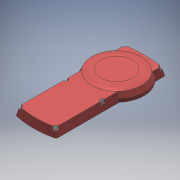
# Autodesk Inventor part: ET8
Saved by Autodesk Inventor 2016 (Build 200138000, 138)
## iProperties
Created: 2016-03-20
Part Number: ET8
Material: Genérico
Document SubType Name: Modeling
Designer: Usuario1
Density: 1 g/cm^3
Appearance: Valor por defecto
Author: Usuario1
Autodesk Inventor part; units mm, degrees
ref_plane "YZ Plane" through (0, 0, 0) normal (1, 0, 0) x (0, 1, 0)
ref_plane "XZ Plane" through (0, 0, 0) normal (0, 1, 0) x (-1, 0, 0)
ref_plane "XY Plane" through (0, 0, 0) normal (0, 0, 1) x (1, 0, 0)
sketch "Boceto1" plane through (0, 0, 0) normal (0, 0, 1) x (1, 0, 0)
  arc A0 (0.1163, -0.2747) -> (3.2914, -0.2747) centre (1.7039, 6.6157) ccw
  arc A1 (3.2914, -0.2747) -> (3.4078, -0.1285) centre (3.2578, -0.1285) ccw
  arc A2 (0, -0.1285) -> (0.1163, -0.2747) centre (0.15, -0.1285) ccw
  circle A3 centre (1.7039, 6.4933) radius 2.0393
  circle A4 centre (0.1483, 3.7581) radius 0.092
  arc A5 (3.2776, 8.8751) -> (0.1302, 8.8751) centre (1.7039, -2.9316) ccw
  arc A6 (3.4078, 8.7264) -> (3.2776, 8.8751) centre (3.2578, 8.7264) ccw
  arc A7 (0.1302, 8.8751) -> (0, 8.7264) centre (0.15, 8.7264) ccw
  line L0 (0, 3.6296) -> (0.16, 3.6296)
  arc A8 (0.16, 3.6296) -> (0.28, 3.7496) centre (0.16, 3.7496) ccw
  line L1 (0.28, 3.7496) -> (0.28, 3.7683)
  arc A9 (0.28, 3.7683) -> (0.16, 3.8883) centre (0.16, 3.7683) ccw
  line L2 (0.16, 3.8883) -> (0, 3.8883)
  circle A10 centre (0.15, 8.7264) radius 0.092
  line L3 (0, 8.5978) -> (0.16, 8.5978)
  line L4 (0.28, 8.8941) -> (0.28, 8.7178)
  arc A11 (0.16, 8.5978) -> (0.28, 8.7178) centre (0.16, 8.7178) ccw
  circle A12 centre (0.15, -0.1285) radius 0.092
  line L5 (0, 0) -> (0.16, 0)
  line L6 (0.28, -0.3104) -> (0.28, -0.12)
  arc A13 (0.28, -0.12) -> (0.16, 0) centre (0.16, -0.12) ccw
  circle A14 centre (3.2594, 3.7581) radius 0.092
  line L7 (3.4078, 3.6296) -> (3.2478, 3.6296)
  arc A15 (3.1278, 3.7496) -> (3.2478, 3.6296) centre (3.2478, 3.7496) ccw
  line L8 (3.1278, 3.7496) -> (3.1278, 3.7683)
  arc A16 (3.2478, 3.8883) -> (3.1278, 3.7683) centre (3.2478, 3.7683) ccw
  line L9 (3.2478, 3.8883) -> (3.4078, 3.8883)
  circle A17 centre (3.2578, 8.7264) radius 0.092
  line L10 (3.4078, 8.5978) -> (3.2478, 8.5978)
  line L11 (3.1278, 8.8941) -> (3.1278, 8.7178)
  arc A18 (3.1278, 8.7178) -> (3.2478, 8.5978) centre (3.2478, 8.7178) ccw
  circle A19 centre (3.2578, -0.1285) radius 0.092
  line L12 (3.4078, 0) -> (3.2478, 0)
  line L13 (3.1278, -0.3104) -> (3.1278, -0.12)
  arc A20 (3.2478, 0) -> (3.1278, -0.12) centre (3.2478, -0.12) ccw
  line L14 (0, 8.7264) -> (0, 7.9849)
  line L15 (3.4078, 8.7264) -> (3.4078, 7.9849)
  line L16 (0, 5.0017) -> (0, -0.1285)
  line L17 (3.4078, -0.1285) -> (3.4078, 5.0017)
  arc A21 (0, 7.9849) -> (0, 5.0017) centre (1.7039, 6.4933) ccw
  arc A22 (3.4078, 5.0017) -> (3.4078, 7.9849) centre (1.7039, 6.4933) ccw
  point P0 (0, 0)
  constraints: 36 end point, 36 point on circle, 23 centre point, 8 point on line
extrude "Extrusión1" add sketch "Boceto1" along normal blind 0.15 contours L6 A13 L5 L16 L0 A8 L1 A9 L2 A21 L14 L3 A11 L4 A5 L11 A18 L10 L15 A22 L17 L9 A16 L8 A15 L7 L12 A20 L13 A0 | A3
sketch "Boceto4" plane through (0, 0, 0) normal (0, 0, -1) x (-1, 0, 0)
  line L0 (0, 3.6296) -> (0, 0) projected
  line L1 (-0.16, 3.6296) -> (0, 3.6296) projected
  arc A0 (-0.28, 3.7496) -> (-0.16, 3.6296) centre (-0.16, 3.7496) ccw projected
  line L2 (-0.28, 3.7683) -> (-0.28, 3.7496) projected
  arc A1 (-0.16, 3.8883) -> (-0.28, 3.7683) centre (-0.16, 3.7683) ccw projected
  line L3 (0, 3.8883) -> (-0.16, 3.8883) projected
  line L4 (0, 5.0017) -> (0, 3.8883) projected
  arc A2 (0, 5.0017) -> (0, 7.9849) centre (-1.7039, 6.4933) ccw projected
  line L5 (0, 8.5978) -> (0, 7.9849) projected
  line L6 (-0.16, 8.5978) -> (0, 8.5978) projected
  arc A3 (-0.28, 8.7178) -> (-0.16, 8.5978) centre (-0.16, 8.7178) ccw projected
  line L7 (-0.28, 8.8941) -> (-0.28, 8.7178) projected
  arc A4 (-0.28, 8.8941) -> (-3.1278, 8.8941) centre (-1.7039, -2.9316) ccw projected
  line L8 (-3.1278, 8.7178) -> (-3.1278, 8.8941) projected
  arc A5 (-3.2478, 8.5978) -> (-3.1278, 8.7178) centre (-3.2478, 8.7178) ccw projected
  line L9 (-3.4078, 8.5978) -> (-3.2478, 8.5978) projected
  line L10 (-3.4078, 7.9849) -> (-3.4078, 8.5978) projected
  arc A6 (-3.4078, 7.9849) -> (-3.4078, 5.0017) centre (-1.7039, 6.4933) ccw projected
  line L11 (-3.4078, 3.8883) -> (-3.4078, 5.0017) projected
  line L12 (-3.2478, 3.8883) -> (-3.4078, 3.8883) projected
  arc A7 (-3.1278, 3.7683) -> (-3.2478, 3.8883) centre (-3.2478, 3.7683) ccw projected
  line L13 (-3.1278, 3.7496) -> (-3.1278, 3.7683) projected
  arc A8 (-3.2478, 3.6296) -> (-3.1278, 3.7496) centre (-3.2478, 3.7496) ccw projected
  line L14 (-3.4078, 3.6296) -> (-3.2478, 3.6296) projected
  line L15 (-3.4078, 0) -> (-3.4078, 3.6296) projected
  line L16 (-3.2478, 0) -> (-3.4078, 0) projected
  arc A9 (-3.1278, -0.12) -> (-3.2478, 0) centre (-3.2478, -0.12) ccw projected
  line L17 (-3.1278, -0.3104) -> (-3.1278, -0.12) projected
  arc A10 (-3.1278, -0.3104) -> (-0.28, -0.3104) centre (-1.7039, 6.6157) ccw projected
  line L18 (-0.28, -0.12) -> (-0.28, -0.3104) projected
  arc A11 (-0.16, 0) -> (-0.28, -0.12) centre (-0.16, -0.12) ccw projected
  line L19 (0, 0) -> (-0.16, 0) projected
  arc A12 (-0.5269, 8.6699) -> (-2.8809, 8.6699) centre (-1.7039, -2.9316) ccw
  arc A13 (-0.5269, 8.6699) -> (-0.25, 8.359) centre (-0.16, 8.7178) ccw
  line L20 (-0.25, 8.359) -> (-0.25, 7.8877)
  arc A14 (-0.25, 5.0988) -> (-0.25, 7.8877) centre (-1.7039, 6.4933) ccw
  line L21 (-0.25, 5.0988) -> (-0.25, 4.1271)
  arc A15 (-0.25, 4.1271) -> (-0.53, 3.7683) centre (-0.16, 3.7683) ccw
  line L22 (-0.53, 3.7683) -> (-0.53, 3.7496)
  arc A16 (-0.53, 3.7496) -> (-0.25, 3.3907) centre (-0.16, 3.7496) ccw
  line L23 (-0.25, 3.3907) -> (-0.25, 0.2389)
  arc A17 (-0.25, 0.2389) -> (-0.5296, -0.1034) centre (-0.16, -0.12) ccw
  arc A18 (-2.8781, -0.1034) -> (-0.5296, -0.1034) centre (-1.7039, 6.6157) ccw
  arc A19 (-2.8781, -0.1034) -> (-3.1578, 0.2389) centre (-3.2478, -0.12) ccw
  line L24 (-3.1578, 0.2389) -> (-3.1578, 3.3907)
  arc A20 (-3.1578, 3.3907) -> (-2.8778, 3.7496) centre (-3.2478, 3.7496) ccw
  line L25 (-2.8778, 3.7496) -> (-2.8778, 3.7683)
  arc A21 (-2.8778, 3.7683) -> (-3.1578, 4.1271) centre (-3.2478, 3.7683) ccw
  line L26 (-3.1578, 4.1271) -> (-3.1578, 5.0988)
  arc A22 (-3.1578, 7.8877) -> (-3.1578, 5.0988) centre (-1.7039, 6.4933) ccw
  line L27 (-3.1578, 7.8877) -> (-3.1578, 8.359)
  arc A23 (-3.1578, 8.359) -> (-2.8809, 8.6699) centre (-3.2478, 8.7178) ccw
  point P0 (0, 0)
  dimension "d10" = 0.25
  constraints: 24 point on circle, 16 end point, 12 centre point, 19 other
  measures "d10" radial gap between concentric circles of A4 A12
extrude "Extrusión4" add sketch "Boceto4" along normal blind 0.52
sketch "Boceto5" plane through (0, 0, 0.15) normal (0, 0, 1) x (1, 0, 0)
  arc A0 (3.2202, 5.0739) -> (3.2202, 7.9126) centre (1.7039, 6.4933) ccw projected
  circle A1 centre (1.7039, 6.4933) radius 2.077
  point P0 (0, 0)
  constraints: 1 coincident, 3 other
extrude "Extrusión5" add sketch "Boceto5" along normal blind 0.15
fillet "Empalme2" radius 2 1 edges at (-0.3731, 6.4933, 0.3)
chamfer "Chaflán12" distance 0.67 angle 15 1 edges at (0, 4.445, 0.15) measured on face at (0, 4.445, -0.35)
chamfer "Chaflán13" distance 0.67 angle 15 1 edges at (0, 1.8148, 0.15) measured on face at (0, 1.8148, -0.35)
chamfer "Chaflán14" distance 0.67 angle 15 1 edges at (1.7039, -0.4552, 0.15) measured on face at (1.7039, -0.4552, -0.35)
chamfer "Chaflán15" distance 0.67 angle 15 1 edges at (3.4078, 1.8148, 0.15) measured on face at (3.4078, 1.8148, -0.35)
chamfer "Chaflán16" distance 0.67 angle 15 1 edges at (3.4078, 4.445, 0.15) measured on face at (3.4078, 4.445, -0.35)
chamfer "Chaflán17" distance 0.67 angle 15 1 edges at (1.7039, 8.9795, 0.15) measured on face at (1.7039, 8.9795, -0.35)
chamfer "Chaflán18" distance 0.67 angle 15 1 edges at (3.4078, 8.2914, 0.15) measured on face at (3.4078, 8.2914, -0.35)
chamfer "Chaflán19" distance 0.67 angle 15 1 edges at (0, 8.2914, 0.15) measured on face at (0, 8.2914, -0.35)
chamfer "Chaflán20" distance 0.4 angle 25 3 edges at (3.3206, 8.0789, 0.15) (3.9684, 6.4933, 0.15) (3.3206, 4.9077, 0.15) measured on face at (3.3206, 8.0789, 0.05) measured on face at (3.3206, 4.9077, 0.05) measured on face at (3.9684, 6.4933, -0.35)
chamfer "Chaflán21" distance 0.4 angle 25 3 edges at (0.0871, 8.0789, 0.15) (-0.5606, 6.4933, 0.15) (0.0871, 4.9077, 0.15) measured on face at (-0.5606, 6.4933, -0.35) measured on face at (0.0871, 8.0789, 0.05) measured on face at (0.0871, 4.9077, 0.05)
sketch "Boceto8" plane through (0, 0, -0.52) normal (0, 0, -1) x (-1, 0, 0)
  arc A0 (-0.5269, 8.6699) -> (-0.25, 8.359) centre (-0.16, 8.7178) ccw projected
  line L0 (-0.25, 8.359) -> (-0.25, 7.8877) projected
  arc A1 (-0.25, 5.0988) -> (-0.25, 7.8877) centre (-1.7039, 6.4933) ccw projected
  line L1 (-0.25, 5.0988) -> (-0.25, 4.1271) projected
  arc A2 (-0.25, 4.1271) -> (-0.53, 3.7683) centre (-0.16, 3.7683) ccw projected
  line L2 (-0.53, 3.7683) -> (-0.53, 3.7496) projected
  arc A3 (-0.53, 3.7496) -> (-0.25, 3.3907) centre (-0.16, 3.7496) ccw projected
  line L3 (-0.25, 3.3907) -> (-0.25, 0.2389) projected
  arc A4 (-0.25, 0.2389) -> (-0.5296, -0.1034) centre (-0.16, -0.12) ccw projected
  arc A5 (-2.8781, -0.1034) -> (-0.5296, -0.1034) centre (-1.7039, 6.6157) ccw projected
  arc A6 (-2.8781, -0.1034) -> (-3.1578, 0.2389) centre (-3.2478, -0.12) ccw projected
  line L4 (-3.1578, 0.2389) -> (-3.1578, 3.3907) projected
  arc A7 (-3.1578, 3.3907) -> (-2.8778, 3.7496) centre (-3.2478, 3.7496) ccw projected
  line L5 (-2.8778, 3.7496) -> (-2.8778, 3.7683) projected
  arc A8 (-2.8778, 3.7683) -> (-3.1578, 4.1271) centre (-3.2478, 3.7683) ccw projected
  line L6 (-3.1578, 4.1271) -> (-3.1578, 5.0988) projected
  arc A9 (-3.1578, 7.8877) -> (-3.1578, 5.0988) centre (-1.7039, 6.4933) ccw projected
  line L7 (-3.1578, 7.8877) -> (-3.1578, 8.359) projected
  arc A10 (-3.1578, 8.359) -> (-2.8809, 8.6699) centre (-3.2478, 8.7178) ccw projected
  arc A11 (-0.5269, 8.6699) -> (-2.8809, 8.6699) centre (-1.7039, -2.9316) ccw projected
  line L8 (0, 0) -> (0, 3.6296) projected
  line L9 (0, 3.6296) -> (-0.16, 3.6296) projected
  arc A12 (-0.28, 3.7496) -> (-0.16, 3.6296) centre (-0.16, 3.7496) ccw projected
  line L10 (-0.28, 3.7496) -> (-0.28, 3.7683) projected
  arc A13 (-0.16, 3.8883) -> (-0.28, 3.7683) centre (-0.16, 3.7683) ccw projected
  line L11 (-0.16, 3.8883) -> (0, 3.8883) projected
  line L12 (0, 3.8883) -> (0, 5.0017) projected
  arc A14 (0, 5.0017) -> (0, 7.9849) centre (-1.7039, 6.4933) ccw projected
  line L13 (0, 7.9849) -> (0, 8.5978) projected
  line L14 (0, 8.5978) -> (-0.16, 8.5978) projected
  arc A15 (-0.28, 8.7178) -> (-0.16, 8.5978) centre (-0.16, 8.7178) ccw projected
  line L15 (-0.28, 8.7178) -> (-0.28, 8.8941) projected
  arc A16 (-0.28, 8.8941) -> (-3.1278, 8.8941) centre (-1.7039, -2.9316) ccw projected
  line L16 (-3.1278, 8.8941) -> (-3.1278, 8.7178) projected
  arc A17 (-3.2478, 8.5978) -> (-3.1278, 8.7178) centre (-3.2478, 8.7178) ccw projected
  line L17 (-3.2478, 8.5978) -> (-3.4078, 8.5978) projected
  line L18 (-3.4078, 8.5978) -> (-3.4078, 7.9849) projected
  arc A18 (-3.4078, 7.9849) -> (-3.4078, 5.0017) centre (-1.7039, 6.4933) ccw projected
  line L19 (-3.4078, 5.0017) -> (-3.4078, 3.8883) projected
  line L20 (-3.4078, 3.8883) -> (-3.2478, 3.8883) projected
  arc A19 (-3.1278, 3.7683) -> (-3.2478, 3.8883) centre (-3.2478, 3.7683) ccw projected
  line L21 (-3.1278, 3.7683) -> (-3.1278, 3.7496) projected
  arc A20 (-3.2478, 3.6296) -> (-3.1278, 3.7496) centre (-3.2478, 3.7496) ccw projected
  line L22 (-3.2478, 3.6296) -> (-3.4078, 3.6296) projected
  line L23 (-3.4078, 3.6296) -> (-3.4078, 0) projected
  line L24 (-3.4078, 0) -> (-3.2478, 0) projected
  arc A21 (-3.1278, -0.12) -> (-3.2478, 0) centre (-3.2478, -0.12) ccw projected
  line L25 (-3.1278, -0.12) -> (-3.1278, -0.3104) projected
  arc A22 (-3.1278, -0.3104) -> (-0.28, -0.3104) centre (-1.7039, 6.6157) ccw projected
  line L26 (-0.28, -0.3104) -> (-0.28, -0.12) projected
  arc A23 (-0.16, 0) -> (-0.28, -0.12) centre (-0.16, -0.12) ccw projected
  line L27 (-0.16, 0) -> (0, 0) projected
  arc A24 (-3.2914, -0.2747) -> (-0.1163, -0.2747) centre (-1.7039, 6.6157) ccw
  arc A25 (-0.1163, -0.2747) -> (0, -0.1285) centre (-0.15, -0.1285) ccw
  arc A26 (-3.4078, -0.1285) -> (-3.2914, -0.2747) centre (-3.2578, -0.1285) ccw
  circle A27 centre (-1.7039, 6.4933) radius 2.0393
  circle A28 centre (-3.2594, 3.7581) radius 0.092
  arc A29 (-0.1302, 8.8751) -> (-3.2776, 8.8751) centre (-1.7039, -2.9316) ccw
  arc A30 (0, 8.7264) -> (-0.1302, 8.8751) centre (-0.15, 8.7264) ccw
  arc A31 (-3.2776, 8.8751) -> (-3.4078, 8.7264) centre (-3.2578, 8.7264) ccw
  line L28 (-3.4078, 3.6296) -> (-3.2478, 3.6296)
  arc A32 (-3.2478, 3.6296) -> (-3.1278, 3.7496) centre (-3.2478, 3.7496) ccw
  line L29 (-3.1278, 3.7496) -> (-3.1278, 3.7683)
  arc A33 (-3.1278, 3.7683) -> (-3.2478, 3.8883) centre (-3.2478, 3.7683) ccw
  line L30 (-3.2478, 3.8883) -> (-3.4078, 3.8883)
  circle A34 centre (-3.2578, 8.7264) radius 0.092
  line L31 (-3.4078, 8.5978) -> (-3.2478, 8.5978)
  line L32 (-3.1278, 8.8941) -> (-3.1278, 8.7178)
  arc A35 (-3.2478, 8.5978) -> (-3.1278, 8.7178) centre (-3.2478, 8.7178) ccw
  circle A36 centre (-3.2578, -0.1285) radius 0.092
  line L33 (-3.4078, 0) -> (-3.2478, 0)
  line L34 (-3.1278, -0.3104) -> (-3.1278, -0.12)
  arc A37 (-3.1278, -0.12) -> (-3.2478, 0) centre (-3.2478, -0.12) ccw
  circle A38 centre (-0.1483, 3.7581) radius 0.092
  line L35 (0, 3.6296) -> (-0.16, 3.6296)
  arc A39 (-0.28, 3.7496) -> (-0.16, 3.6296) centre (-0.16, 3.7496) ccw
  line L36 (-0.28, 3.7496) -> (-0.28, 3.7683)
  arc A40 (-0.16, 3.8883) -> (-0.28, 3.7683) centre (-0.16, 3.7683) ccw
  line L37 (-0.16, 3.8883) -> (0, 3.8883)
  circle A41 centre (-0.15, 8.7264) radius 0.092
  line L38 (0, 8.5978) -> (-0.16, 8.5978)
  line L39 (-0.28, 8.8941) -> (-0.28, 8.7178)
  arc A42 (-0.28, 8.7178) -> (-0.16, 8.5978) centre (-0.16, 8.7178) ccw
  circle A43 centre (-0.15, -0.1285) radius 0.092
  line L40 (0, 0) -> (-0.16, 0)
  line L41 (-0.28, -0.3104) -> (-0.28, -0.12)
  arc A44 (-0.16, 0) -> (-0.28, -0.12) centre (-0.16, -0.12) ccw
  line L42 (-3.4078, 8.7264) -> (-3.4078, 7.9849)
  line L43 (0, 8.7264) -> (0, 7.9849)
  line L44 (-3.4078, 5.0017) -> (-3.4078, -0.1285)
  line L45 (0, -0.1285) -> (0, 5.0017)
  arc A45 (-3.4078, 7.9849) -> (-3.4078, 5.0017) centre (-1.7039, 6.4933) ccw
  arc A46 (0, 5.0017) -> (0, 7.9849) centre (-1.7039, 6.4933) ccw
  point P0 (0, 0)
  constraints: 36 end point, 36 point on circle, 23 centre point, 8 point on line
extrude "Extrusión8" add sketch "Boceto8" against normal blind 0.4 contours L45 A25 A24 L26 A23 L27 | L9 A12 L10 A13 L11 L45 | A24 A26 L44 L24 A21 L25 | L14 A15 L15 A29 A30 L43 | L44 L20 A19 L21 A20 L22 | L16 A17 L17 L42 A31 A29 | A28 | A34 | A36 | A38 | A41 | A43
chamfer "Chaflán22" distance 0.4 angle 15 1 edges at (3.4078, 3.7589, -0.12) measured on face at (3.4078, 3.7589, -0.22)
chamfer "Chaflán23" distance 0.4 angle 15 3 edges at (3.4078, 8.6621, -0.12) (3.3706, 8.8252, -0.12) (3.2027, 8.8848, -0.12) measured on face at (3.1901, 8.7856, -0.12) measured on face at (3.3706, 8.8252, -0.22) measured on face at (3.4078, 8.6621, -0.22)
chamfer "Chaflán24" distance 0.4 angle 15 3 edges at (0.2051, 8.8848, -0.12) (0.0371, 8.8252, -0.12) (0, 8.6621, -0.12) measured on face at (0.1, 8.6621, -0.12) measured on face at (0.0371, 8.8252, -0.22) measured on face at (0.2051, 8.8848, -0.22)
chamfer "Chaflán25" distance 0.4 angle 15 1 edges at (0, 3.7589, -0.12) measured on face at (0, 3.7589, -0.22)
chamfer "Chaflán26" distance 0.4 angle 15 3 edges at (3.3751, -0.2219, -0.12) (3.4078, -0.0643, -0.12) (3.2097, -0.293, -0.12) measured on face at (3.2097, -0.293, -0.22) measured on face at (3.3751, -0.2219, -0.22) measured on face at (3.4078, -0.0643, -0.22)
chamfer "Chaflán27" distance 0.4 angle 15 3 edges at (0.0326, -0.2219, -0.12) (0.1981, -0.293, -0.12) (0, -0.0643, -0.12) measured on face at (0.1981, -0.293, -0.22) measured on face at (0.0326, -0.2219, -0.22) measured on face at (0, -0.0643, -0.22)
sketch "Boceto9" plane through (0, 0, -0.52) normal (0, 0, -1) x (-1, 0, 0)
  arc A0 (-0.5269, 8.6699) -> (-0.25, 8.359) centre (-0.16, 8.7178) ccw projected
  line L0 (-0.25, 8.359) -> (-0.25, 7.8877) projected
  arc A1 (-0.25, 5.0988) -> (-0.25, 7.8877) centre (-1.7039, 6.4933) ccw projected
  line L1 (-0.25, 5.0988) -> (-0.25, 4.1271) projected
  arc A2 (-0.25, 4.1271) -> (-0.53, 3.7683) centre (-0.16, 3.7683) ccw projected
  line L2 (-0.53, 3.7683) -> (-0.53, 3.7496) projected
  arc A3 (-0.53, 3.7496) -> (-0.25, 3.3907) centre (-0.16, 3.7496) ccw projected
  line L3 (-0.25, 3.3907) -> (-0.25, 0.2389) projected
  arc A4 (-0.25, 0.2389) -> (-0.5296, -0.1034) centre (-0.16, -0.12) ccw projected
  arc A5 (-2.8781, -0.1034) -> (-0.5296, -0.1034) centre (-1.7039, 6.6157) ccw projected
  arc A6 (-2.8781, -0.1034) -> (-3.1578, 0.2389) centre (-3.2478, -0.12) ccw projected
  line L4 (-3.1578, 0.2389) -> (-3.1578, 3.3907) projected
  arc A7 (-3.1578, 3.3907) -> (-2.8778, 3.7496) centre (-3.2478, 3.7496) ccw projected
  line L5 (-2.8778, 3.7496) -> (-2.8778, 3.7683) projected
  arc A8 (-2.8778, 3.7683) -> (-3.1578, 4.1271) centre (-3.2478, 3.7683) ccw projected
  line L6 (-3.1578, 4.1271) -> (-3.1578, 5.0988) projected
  arc A9 (-3.1578, 7.8877) -> (-3.1578, 5.0988) centre (-1.7039, 6.4933) ccw projected
  line L7 (-3.1578, 7.8877) -> (-3.1578, 8.359) projected
  arc A10 (-3.1578, 8.359) -> (-2.8809, 8.6699) centre (-3.2478, 8.7178) ccw projected
  arc A11 (-0.5269, 8.6699) -> (-2.8809, 8.6699) centre (-1.7039, -2.9316) ccw projected
  line L8 (0, -0.1285) -> (0, 5.0017) projected
  arc A12 (0, 5.0017) -> (0, 7.9849) centre (-1.7039, 6.4933) ccw projected
  line L9 (0, 7.9849) -> (0, 8.7264) projected
  arc A13 (0, 8.7264) -> (-0.1302, 8.8751) centre (-0.15, 8.7264) ccw projected
  arc A14 (-0.1302, 8.8751) -> (-0.28, 8.8941) centre (-1.7039, -2.9316) ccw projected
  arc A15 (-0.28, 8.8941) -> (-3.1278, 8.8941) centre (-1.7039, -2.9316) ccw projected
  arc A16 (-3.1278, 8.8941) -> (-3.2776, 8.8751) centre (-1.7039, -2.9316) ccw projected
  arc A17 (-3.2776, 8.8751) -> (-3.4078, 8.7264) centre (-3.2578, 8.7264) ccw projected
  line L10 (-3.4078, 8.7264) -> (-3.4078, 7.9849) projected
  arc A18 (-3.4078, 7.9849) -> (-3.4078, 5.0017) centre (-1.7039, 6.4933) ccw projected
  line L11 (-3.4078, 5.0017) -> (-3.4078, -0.1285) projected
  arc A19 (-3.4078, -0.1285) -> (-3.2914, -0.2747) centre (-3.2578, -0.1285) ccw projected
  arc A20 (-3.2914, -0.2747) -> (-0.1163, -0.2747) centre (-1.7039, 6.6157) ccw projected
  arc A21 (-0.1163, -0.2747) -> (0, -0.1285) centre (-0.15, -0.1285) ccw projected
  line L12 (-0.15, 4.0381) -> (-0.15, 5.0592)
  arc A22 (-0.15, 5.0592) -> (-0.15, 7.9274) centre (-1.7039, 6.4933) ccw
  line L13 (-0.15, 7.9274) -> (-0.15, 8.448)
  arc A23 (-0.4267, 8.7599) -> (-0.15, 8.448) centre (-0.16, 8.7178) ccw
  arc A24 (-0.4267, 8.7599) -> (-2.9811, 8.7599) centre (-1.7039, -2.9316) ccw
  arc A25 (-3.2578, 8.448) -> (-2.9811, 8.7599) centre (-3.2478, 8.7178) ccw
  line L14 (-3.2578, 8.448) -> (-3.2578, 7.9274)
  arc A26 (-3.2578, 7.9274) -> (-3.2578, 5.0592) centre (-1.7039, 6.4933) ccw
  line L15 (-3.2578, 5.0592) -> (-3.2578, 4.0381)
  arc A27 (-2.9778, 3.7683) -> (-3.2578, 4.0381) centre (-3.2478, 3.7683) ccw
  line L16 (-2.9778, 3.7683) -> (-2.9778, 3.7496)
  arc A28 (-3.2578, 3.4798) -> (-2.9778, 3.7496) centre (-3.2478, 3.7496) ccw
  line L17 (-3.2578, 3.4798) -> (-3.2578, 0.1498)
  arc A29 (-2.9858, -0.1855) -> (-3.2578, 0.1498) centre (-3.2478, -0.12) ccw
  arc A30 (-2.9858, -0.1855) -> (-0.4219, -0.1855) centre (-1.7039, 6.6157) ccw
  arc A31 (-0.15, 0.1498) -> (-0.4219, -0.1855) centre (-0.16, -0.12) ccw
  line L18 (-0.15, 0.1498) -> (-0.15, 3.4798)
  arc A32 (-0.43, 3.7496) -> (-0.15, 3.4798) centre (-0.16, 3.7496) ccw
  line L19 (-0.43, 3.7496) -> (-0.43, 3.7683)
  arc A33 (-0.15, 4.0381) -> (-0.43, 3.7683) centre (-0.16, 3.7683) ccw
  point P0 (0, 0)
  dimension "d101" = 0.1
  constraints: 24 point on circle, 16 end point, 12 centre point, 19 other
  measures "d101" distance between parallel lines of L1 L12
extrude "Extrusión9" cut sketch "Boceto9" against normal blind 0.3 contours A33 L19 A32 L18 A31 A30 A29 L17 A28 L16 A27 L15 A26 L14 A25 A24 A23 L13 A22 L12
sketch "Boceto10" plane through (0, 0, -0.12) normal (0, 0, 1) x (1, 0, 0)
  line L0 (0.1072, -0.1285) -> (0.1072, 0) projected
  arc A0 (0.1072, -0.1285) -> (0.1404, -0.1703) centre (0.15, -0.1285) ccw projected
  arc A1 (0.1404, -0.1703) -> (0.28, -0.2009) centre (1.7039, 6.6157) ccw projected
  line L1 (0.28, -0.12) -> (0.28, -0.2009) projected
  arc A2 (0.28, -0.12) -> (0.16, 0) centre (0.16, -0.12) ccw projected
  line L2 (0.1072, 0) -> (0.16, 0) projected
  line L3 (0.1072, 3.6296) -> (0.1072, 3.8883) projected
  line L4 (0.16, 3.6296) -> (0.1072, 3.6296) projected
  arc A3 (0.16, 3.6296) -> (0.28, 3.7496) centre (0.16, 3.7496) ccw projected
  line L5 (0.28, 3.7683) -> (0.28, 3.7496) projected
  arc A4 (0.28, 3.7683) -> (0.16, 3.8883) centre (0.16, 3.7683) ccw projected
  line L6 (0.1072, 3.8883) -> (0.16, 3.8883) projected
  line L7 (3.3006, 3.8883) -> (3.3006, 3.6296) projected
  line L8 (3.2478, 3.8883) -> (3.3006, 3.8883) projected
  arc A5 (3.2478, 3.8883) -> (3.1278, 3.7683) centre (3.2478, 3.7683) ccw projected
  line L9 (3.1278, 3.7496) -> (3.1278, 3.7683) projected
  arc A6 (3.1278, 3.7496) -> (3.2478, 3.6296) centre (3.2478, 3.7496) ccw projected
  line L10 (3.3006, 3.6296) -> (3.2478, 3.6296) projected
  arc A7 (3.1278, -0.2009) -> (3.2674, -0.1703) centre (1.7039, 6.6157) ccw projected
  arc A8 (3.2674, -0.1703) -> (3.3006, -0.1285) centre (3.2578, -0.1285) ccw projected
  line L11 (3.3006, 0) -> (3.3006, -0.1285) projected
  line L12 (3.2478, 0) -> (3.3006, 0) projected
  arc A9 (3.2478, 0) -> (3.1278, -0.12) centre (3.2478, -0.12) ccw projected
  line L13 (3.1278, -0.2009) -> (3.1278, -0.12) projected
  line L14 (3.3006, 8.7264) -> (3.3006, 8.5978) projected
  arc A10 (3.3006, 8.7264) -> (3.2634, 8.7688) centre (3.2578, 8.7264) ccw projected
  arc A11 (3.2634, 8.7688) -> (3.1278, 8.7861) centre (1.7039, -2.9316) ccw projected
  line L15 (3.1278, 8.7178) -> (3.1278, 8.7861) projected
  arc A12 (3.1278, 8.7178) -> (3.2478, 8.5978) centre (3.2478, 8.7178) ccw projected
  line L16 (3.3006, 8.5978) -> (3.2478, 8.5978) projected
  arc A13 (0.28, 8.7861) -> (0.1443, 8.7688) centre (1.7039, -2.9316) ccw projected
  arc A14 (0.1443, 8.7688) -> (0.1072, 8.7264) centre (0.15, 8.7264) ccw projected
  line L17 (0.1072, 8.5978) -> (0.1072, 8.7264) projected
  line L18 (0.16, 8.5978) -> (0.1072, 8.5978) projected
  arc A15 (0.16, 8.5978) -> (0.28, 8.7178) centre (0.16, 8.7178) ccw projected
  line L19 (0.28, 8.7861) -> (0.28, 8.7178) projected
  arc A16 (0.28, 8.7861) -> (0.1443, 8.7688) centre (1.7039, -2.9316) ccw projected
  line L20 (0.1072, 3.6296) -> (0.1072, 3.8883) projected
  circle A17 centre (0.1952, 3.7589) radius 0.075
  line L21 (0.1072, -0.1285) -> (0.1072, 0) projected
  circle A18 centre (0.1952, -0.0989) radius 0.075
  line L22 (0.1072, 8.5978) -> (0.1072, 8.7264) projected
  circle A19 centre (0.1952, 8.6949) radius 0.075
  circle A20 centre (1.7039, 6.4933) radius 1.317 projected
  circle A21 centre (3.2126, 3.7589) radius 0.075
  circle A22 centre (3.2126, -0.0989) radius 0.075
  circle A23 centre (3.2126, 8.6949) radius 0.075
  point P0 (0, 0)
  dimension "d104" = 0.15
  dimension "d105" = 0.15
  dimension "d106" = 0.15
  constraints: 6 centre point
  measures "d104" diameter of A17
  measures "d105" diameter of A18
  measures "d106" diameter of A19
extrude "Extrusión10" cut sketch "Boceto10" against normal blind 10 contours A17 | A18 | A19 | A21 | A22 | A23
sketch "Boceto11" plane through (0, 0, 0.15) normal (0, 0, 1) x (1, 0, 0)
  arc A0 (0.28, -0.12) -> (0.1795, -0.0016) centre (0.16, -0.12) ccw projected
  line L0 (0.1795, 7.9055) -> (0.1795, 8.5994) projected
  arc A1 (0.1795, 7.9055) -> (0.1795, 5.081) centre (1.7039, 6.4933) ccw projected
  line L1 (0.1795, 3.8867) -> (0.1795, 5.081) projected
  arc A2 (0.28, 3.7683) -> (0.1795, 3.8867) centre (0.16, 3.7683) ccw projected
  line L2 (0.28, 3.7683) -> (0.28, 3.7496) projected
  arc A3 (0.1795, 3.6312) -> (0.28, 3.7496) centre (0.16, 3.7496) ccw projected
  line L3 (0.1795, -0.0016) -> (0.1795, 3.6312) projected
  arc A4 (0.28, -0.12) -> (0.1795, -0.0016) centre (0.16, -0.12) ccw projected
  line L4 (0.28, -0.12) -> (0.28, -0.127) projected
  arc A5 (0.28, -0.127) -> (3.1278, -0.127) centre (1.7039, 6.6157) ccw projected
  line L5 (3.1278, -0.127) -> (3.1278, -0.12) projected
  arc A6 (3.2282, -0.0016) -> (3.1278, -0.12) centre (3.2478, -0.12) ccw projected
  line L6 (3.2282, 3.6312) -> (3.2282, -0.0016) projected
  arc A7 (3.1278, 3.7496) -> (3.2282, 3.6312) centre (3.2478, 3.7496) ccw projected
  line L7 (3.1278, 3.7496) -> (3.1278, 3.7683) projected
  arc A8 (3.2282, 3.8867) -> (3.1278, 3.7683) centre (3.2478, 3.7683) ccw projected
  line L8 (3.2282, 5.081) -> (3.2282, 3.8867) projected
  arc A9 (3.2282, 5.081) -> (3.2282, 7.9055) centre (1.7039, 6.4933) ccw projected
  line L9 (3.2282, 8.5994) -> (3.2282, 7.9055) projected
  arc A10 (3.1278, 8.7132) -> (3.2282, 8.5994) centre (3.2478, 8.7178) ccw projected
  arc A11 (3.1278, 8.7132) -> (0.2799, 8.7132) centre (1.7039, -2.9316) ccw projected
  arc A12 (0.1795, 8.5994) -> (0.2799, 8.7132) centre (0.16, 8.7178) ccw projected
  circle A13 centre (1.7039, 6.4933) radius 2.077 projected
  arc A14 (0.38, -0.12) -> (0.1958, 0.0971) centre (0.16, -0.12) ccw
  line L10 (0.1795, 3.6312) -> (0.1795, 3.5812)
  line L11 (0.1795, -0.0016) -> (0.1795, 3.6312) projected
  line L12 (0.1795, 3.8867) -> (0.1795, 3.9367)
  arc A15 (0.1795, 3.5812) -> (0.1795, 3.9367) centre (0.1795, 3.7589) ccw
  line L13 (0.1795, 3.5812) -> (0.0733, 3.5812)
  line L14 (0.0733, 3.5812) -> (0.0733, 3.9367)
  line L15 (0.0733, 3.9367) -> (0.1795, 3.9367)
  line L16 (0.1958, 0.0971) -> (0.0733, 0.0971)
  line L17 (0.0733, 0.0971) -> (0.0733, -0.2029)
  line L18 (0.0733, -0.2029) -> (0.38, -0.2029)
  line L19 (0.38, -0.2029) -> (0.38, -0.12)
  circle A16 centre (0.1952, 8.6949) radius 0.075 projected
  line L20 (0.1952, 8.5199) -> (-0.0415, 8.5199)
  line L21 (0.3702, 8.6949) -> (0.3702, 9.0015)
  line L22 (0.3702, 9.0015) -> (-0.0415, 9.0015)
  line L23 (-0.0415, 9.0015) -> (-0.0415, 8.5199)
  arc A17 (0.1952, 8.5199) -> (0.3702, 8.6949) centre (0.1952, 8.6949) ccw
  arc A18 (0.28, -0.127) -> (3.1278, -0.127) centre (1.7039, 6.6157) ccw projected
  arc A19 (3.212, 0.0971) -> (3.0278, -0.12) centre (3.2478, -0.12) ccw
  arc A20 (3.2282, 3.9367) -> (3.2282, 3.5812) centre (3.2282, 3.7589) ccw
  line L24 (3.2282, 3.5812) -> (3.3345, 3.5812)
  line L25 (3.3345, 3.5812) -> (3.3345, 3.9367)
  line L26 (3.3345, 3.9367) -> (3.2282, 3.9367)
  line L27 (3.212, 0.0971) -> (3.3345, 0.0971)
  line L28 (3.3345, 0.0971) -> (3.3345, -0.2029)
  line L29 (3.3345, -0.2029) -> (3.0278, -0.2029)
  line L30 (3.2126, 8.5199) -> (3.4492, 8.5199)
  line L31 (3.0376, 8.6949) -> (3.0376, 9.0015)
  line L32 (3.0376, 9.0015) -> (3.4492, 9.0015)
  line L33 (3.4492, 9.0015) -> (3.4492, 8.5199)
  arc A21 (3.0376, 8.6949) -> (3.2126, 8.5199) centre (3.2126, 8.6949) ccw
  line L34 (3.0278, -0.12) -> (3.0278, -0.2029)
  point P0 (0, 0)
  dimension "d109" = 0.1
  dimension "d110" = 0.05
  dimension "d112" = 0.05
  constraints: 48 end point, 12 point on circle, 7 perpendicular, 6 centre point, 6 point on line, 2 horizontal, 2 vertical
  measures "d109" radial gap between concentric circles of A0 A14
  measures "d110" distance of L3.end L10.end
  measures "d112" distance of L1.start L12.end
extrude "Extrusión11" cut sketch "Boceto11" against normal blind 0.27 contours L4 A5 L19 L18 L17 L16 L3 A0 | A0 L3 L16 A14 L19 A5 L4 | L13 L14 L15 L1 A2 L2 A3 L3 | L3 A3 L2 A2 L1 A15 | L34 A19 L27 L6 A6 L5 A5 | A5 L5 A6 L6 L27 L28 L29 L34 | L20 L23 L22 L21 A11 A12 L0 | L0 A12 A11 L21 A17 L20 | L26 L25 L24 L6 A7 L7 A8 L8 | L8 A8 L7 A7 L6 A20 | L30 A21 L31 A11 A10 L9 | L9 A10 A11 L31 L32 L33 L30
